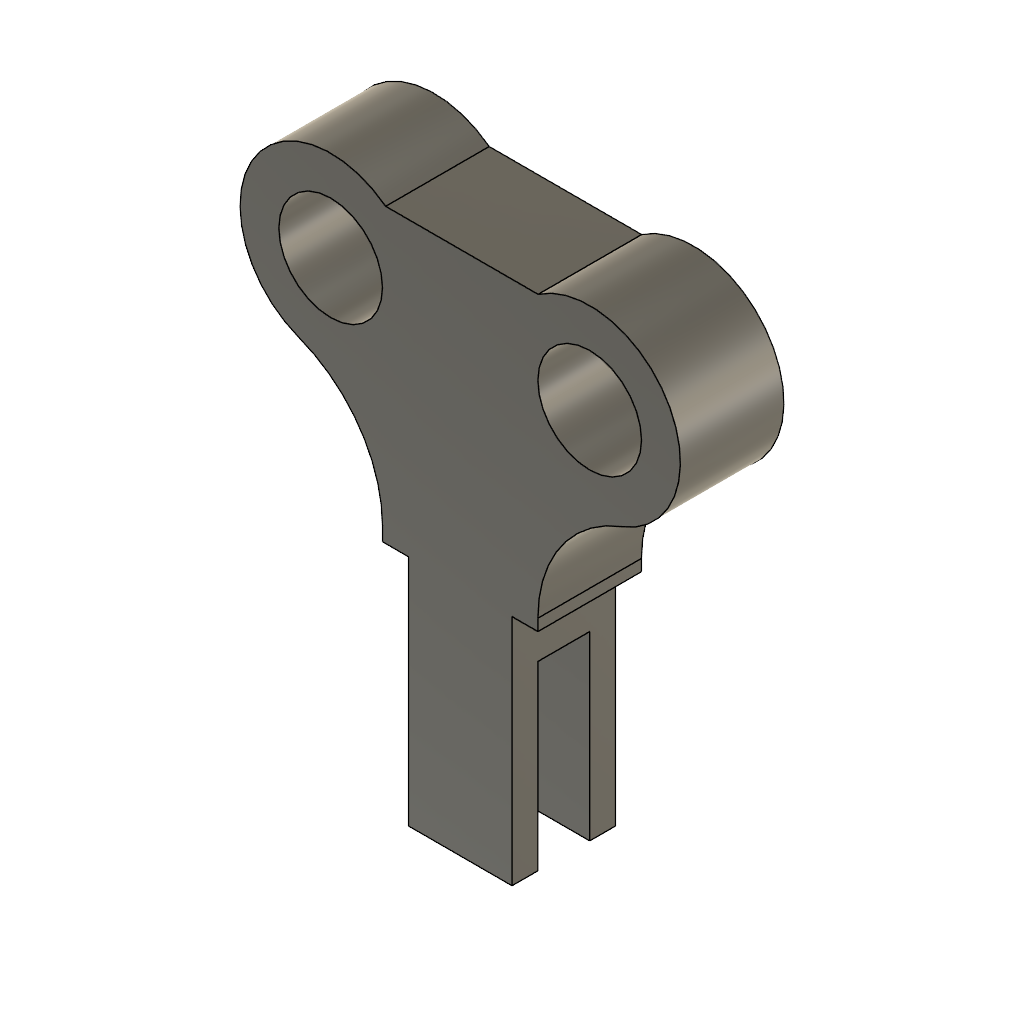
exercise 8 (Autodesk Fusion 360 design; units mm, degrees)
part number: 2026-10-04-11-06-58-206
Autodesk Fusion 360 part; units mm, degrees
sketch "Sketch1" plane through (0, 0, 0) normal (0, 1, 0) x (1, 0, 0)
  circle A0 centre (-35.4096, -0.4721) radius 10
  circle A1 centre (14.5882, 0.0008) radius 10
  line L0 (-0.4096, 42) -> (-0.4096, 87)
  line L1 (-20.4096, 87) -> (-20.4096, 42)
  line L2 (-25.429, 39.2855) -> (-25.429, 42)
  line L3 (4.5904, 39.7649) -> (4.5904, 42)
  line L4 (-20.4096, 42) -> (-25.429, 42)
  line L5 (-25.429, 42) -> (-20.4096, 42)
  line L6 (-0.4096, 42) -> (4.5904, 42)
  arc A2 (4.6294, -14.3892) -> (20.7656, 16.3743) centre (14.5882, 0.0008) ccw
  arc A3 (-41.594, 15.8987) -> (-24.8, -14.3892) centre (-35.4096, -0.4721) ccw
  arc A4 (-41.594, 15.8987) -> (-25.429, 39.2855) centre (-50.429, 39.2855) ccw
  arc A5 (4.5904, 39.7649) -> (20.7656, 16.3743) centre (29.5904, 39.7649) ccw
  line L7 (-24.8, -14.3892) -> (4.6294, -14.3892)
  line L8 (-20.4096, 87) -> (-0.4096, 87)
  dimension "d1" = 50
  dimension "d2" = 20
  dimension "d3" = 20
  dimension "d4" = 35
  dimension "d5" = 35
  dimension "d9" = 20
  dimension "d10" = 45
  dimension "d11" = 15
  dimension "d16" = 25
  dimension "d17" = 25
  constraint concentric A0 A3
  constraint concentric A1 A2
  constraint vertical L0
  constraint vertical L1
  constraint perpendicular L2 L4
  constraint perpendicular L3 L6
  constraint collinear L5 L6
  constraint tangent A3 A4
  constraint tangent L2 A4
  constraint tangent L3 A5
  constraint tangent A2 A5
  constraint horizontal L7
  constraint perpendicular L0 L8
  measures "d1" distance of A0.centre A1.centre
  measures "d2" diameter of A0
  measures "d3" diameter of A1
  measures "d4" diameter of A3
  measures "d5" diameter of A2
  measures "d9" distance of L1.end L0.start
  measures "d10" distance of L1.end L1.start
  measures "d11" horizontal distance of A0.centre L1.end
  measures "d16" radius of A4
  measures "d17" radius of A5
extrude "Extrude1" add sketch "Sketch1" along normal blind 20
sketch "Sketch2" plane through (-0.4096, 0, 0) normal (1, 0, 0) x (0, 1, 0)
  line L0 (0, -42) -> (0, -87)
  line L1 (0, -87) -> (20, -87)
  line L2 (20, -87) -> (20, -42)
  line L3 (20, -42) -> (0, -42)
  line L4 (5, -52) -> (15, -52)
  line L5 (15, -52) -> (15, -87)
  line L6 (15, -87) -> (5, -87)
  line L7 (5, -87) -> (5, -52)
  dimension "d26" = 10
  dimension "d27" = 35
  constraint horizontal L4
  constraint vertical L5
  constraint horizontal L6
  constraint vertical L7
  constraint coincident L1.end L6
  measures "d26" distance of L4.start L4.end
  measures "d27" distance of L4.start L6.end
extrude "Extrude2" cut sketch "Sketch2" against normal blind 47.149 contours L1 L4 L5 L6 L7
